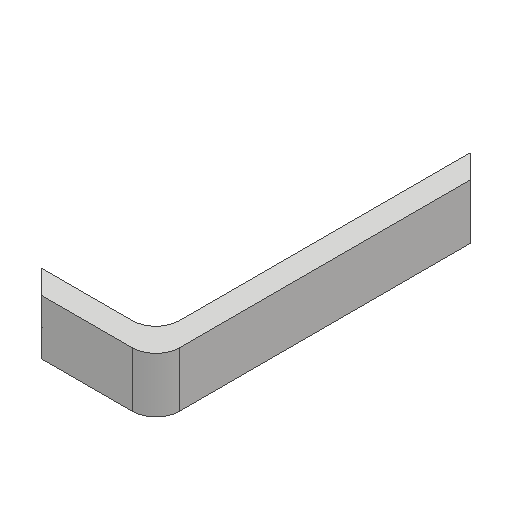
# Autodesk Inventor part: 3DP_PLA_Back_motor_clamp_hole_plug
Saved by Autodesk Inventor 2025 (Build 290162010, 162A)
## iProperties
Created: 2016-05-02
Part Number: 3DP_PLA_Back_motor_clamp_hole_plug
Material: Ogólny
Document SubType Name: Modeling
Designer: Andrzej
Density: 1 g/cm^3
Appearance: Domyślna
Mass: 1.113 g
Surface Area: 11.0167 cm^2
Volume: 1.113 cm^3
Author: Andrzej
Autodesk Inventor part; units mm, degrees
ref_plane "YZ Plane" through (0, 0, 0) normal (1, 0, 0) x (0, 1, 0)
ref_plane "XZ Plane" through (0, 0, 0) normal (0, 1, 0) x (-1, 0, 0)
ref_plane "XY Plane" through (0, 0, 0) normal (0, 0, 1) x (1, 0, 0)
sketch "Szkic1" plane through (0, 0, 0) normal (0, 0, 1) x (1, 0, 0)
  line L0 (-6.6672, -4.667) -> (7.8328, -4.667)
  line L1 (7.8328, -4.667) -> (7.8328, 35.333)
  line L2 (7.8328, 35.333) -> (4.8328, 35.333)
  line L3 (4.8328, 35.333) -> (4.8328, -1.667)
  line L4 (4.8328, -1.667) -> (-6.6672, -1.667)
  line L5 (-6.6672, -1.667) -> (-6.6672, -4.667)
  point P0 (0, 0)
  dimension "d0" = 14.5
  dimension "d1" = 40
  dimension "d3" = 37
  dimension "d8" = 3
  constraints: 12 end point, 4 perpendicular, 1 horizontal, 1 vertical
  measures "d0" distance of L0.start L0.end
  measures "d1" distance of L0.end L1.end
  measures "d3" distance of L2.end L3.end
  measures "d8" distance between parallel lines of L1 L3
extrude "Wyciągnięcie proste1" add sketch "Szkic1" along normal blind 7
fillet "Zaokrąglenie1" radius 3 2 edges at (7.8328, -4.667, 3.5) (4.8328, -1.667, 3.5)
sketch "Szkic2" plane through (0, 0, 7) normal (0, 0, 1) x (1, 0, 0)
  arc A0 (4.8328, -4.667) -> (7.8328, -1.667) centre (4.8328, -1.667) ccw projected
  line L0 (7.8328, -1.667) -> (7.8328, 35.333) projected
  line L1 (7.8328, 35.333) -> (4.8328, 35.333) projected
  line L2 (4.8328, 35.333) -> (4.8328, 1.333) projected
  arc A1 (1.8328, -1.667) -> (4.8328, 1.333) centre (1.8328, 1.333) ccw projected
  line L3 (1.8328, -1.667) -> (-6.6672, -1.667) projected
  line L4 (-6.6672, -1.667) -> (-6.6672, -4.667) projected
  line L5 (-6.6672, -4.667) -> (4.8328, -4.667) projected
  line L6 (-6.6672, -4.667) -> (-9.6672, -1.667)
  line L7 (-6.6672, -4.667) -> (5.1638, -4.667) construction
  line L8 (1.8328, -1.667) -> (-6.6672, -1.667) projected
  line L9 (-6.6672, -1.667) -> (-9.6672, -1.667)
  line L10 (7.8328, 35.333) -> (4.8328, 38.333)
  line L11 (7.8328, 35.333) -> (17.4618, 35.333) construction
  line L12 (4.8328, 35.333) -> (4.8328, 38.333)
  point P0 (0, 0)
  dimension "d13" = 135
  dimension "d15" = 135
  constraints: 12 end point, 2 horizontal, 1 collinear, 1 vertical
  measures "d13" angle of L7 L6
  measures "d15" angle of L11 L10
extrude "Wyciągnięcie proste2" add sketch "Szkic2" against normal blind 3.5 contours L6 L9 L4 | L1 L12 L10
